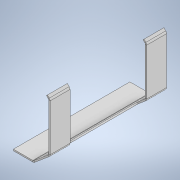
# Autodesk Inventor part: Trasera
Saved by Autodesk Inventor 2021 (Build 250183000, 183)
## iProperties
Created: 2021-07-21
Part Number: Trasera
Material: Generic
Document SubType Name: Sheet Metal
Designer: admin
Density: 1 g/cm^3
Sheet Metal Rule: Por defecto_mm
Appearance: Default
Flat Pattern Width: 32.5 cm
Flat Pattern Length: 41 cm
Flat Pattern Area: 1332.5 cm^2
Sheet Metal Width: 0.325 m
Sheet Metal Length: 0.410 m
Sheet Metal Area: 0.133 m^2
Author: admin
Autodesk Inventor part; units mm, degrees
ref_plane "YZ Plane" through (0, 0, 0) normal (1, 0, 0) x (0, 1, 0)
ref_plane "XZ Plane" through (0, 0, 0) normal (0, 1, 0) x (-1, 0, 0)
ref_plane "XY Plane" through (0, 0, 0) normal (0, 0, 1) x (1, 0, 0)
sketch "Boceto1" plane through (0, 0, 0) normal (0, 1, 0) x (-1, 0, 0)
  line L0 (162.5, 205) -> (-162.5, 205)
  line L1 (-162.5, -205) -> (162.5, -205)
  line L2 (162.5, -205) -> (162.5, 205)
  line L3 (162.5, 205) -> (-162.5, -205) construction
  line L4 (-162.5, 205) -> (162.5, -205) construction
  line L5 (-162.5, -205) -> (-162.5, -135)
  line L6 (-162.5, 205) -> (-162.5, 135)
  line L7 (-162.5, 0) -> (57.5, 0)
  line L8 (-162.5, 135) -> (57.5, 135)
  line L9 (57.5, 135) -> (57.5, -135)
  line L10 (57.5, -135) -> (-162.5, -135)
  line L11 (-162.5, 205) -> (-162.5, 135)
  line L12 (-162.5, -135) -> (-162.5, -205)
  point P0 (0, 0)
  dimension "d0" = 325
  dimension "d1" = 410
  dimension "d24" = 70
  dimension "d25" = 70
  dimension "d26" = 220
  constraints: 26 end point, 4 parallel, 2 horizontal, 2 midpoint, 2 perpendicular
  measures "d0" distance of L1.end L1.start
  measures "d1" distance of L1.start L0.end
  measures "d24" distance of L1.start L5.end
  measures "d25" distance of L6.end L0.end
  measures "d26" distance of L7.start L7.end
extrude "Placa1" add sketch "Boceto1" along normal blind 5
sketch "Boceto3" plane through (0, 5, 0) normal (0, 1, 0) x (1, 0, 0)
  line L0 (-162.5, 205) -> (162.5, 205) projected
  line L1 (-162.5, 205) -> (-91.5, 205)
  line L2 (-91.5, 205) -> (-19.5, 205)
  line L3 (-19.5, 205) -> (150.5, 205)
  line L4 (150.5, 205) -> (150.5, -205) construction
  line L5 (162.5, -205) -> (-162.5, -205) construction
  line L6 (-19.5, 205) -> (-19.5, -205) construction
  line L7 (-91.5, 205) -> (-91.5, -205) construction
  point P0 (0, 0)
  dimension "d27" = 71
  dimension "d28" = 72
  dimension "d29" = 170
  constraints: 12 end point, 5 point on line, 2 vertical, 1 perpendicular
  measures "d27" distance of L0.start L1.end
  measures "d28" distance of L1.end L2.end
  measures "d29" distance of L2.end L3.end
fold "Pliegue4" angle 45 bend radius 5 thickness 5 k factor 0.44 line from (150.5, 5, -205) to (150.5, 5, 205) line at bend centre moving side (1, 0, 0) folds toward (0, 1, 0)
fold "Pliegue5" angle 50 bend radius 5 thickness 5 k factor 0.44 line from (-19.5, 5, -205) to (-19.5, 5, 205) line at bend centre moving side (1, 0, 0) folds toward (0, 1, 0)
fold "Pliegue6" angle 40 bend radius 5 thickness 5 k factor 0.44 line from (-91.5, 5, -205) to (-91.5, 5, 205) line at bend centre moving side (1, 0, 0) folds toward (0, 1, 0)
equation "\"d2\" = Thickness"
equation "\"d30\" = BendReliefWidth"
equation "\"d31\" = BendReliefDepth"
equation "\"d32\" = MinimumRemnant"
equation "\"d33\" = TransitionRadius"
equation "\"d35\" = BendRadius"
equation "\"d36\" = BendReliefWidth"
equation "\"d37\" = BendReliefDepth"
equation "\"d38\" = MinimumRemnant"
equation "\"d39\" = TransitionRadius"
equation "\"d41\" = BendRadius"
equation "\"d42\" = BendReliefWidth"
equation "\"d43\" = BendReliefDepth"
equation "\"d44\" = MinimumRemnant"
equation "\"d45\" = TransitionRadius"
equation "\"d47\" = BendRadius"
equation "\"BendRadius\" = Thickness"
equation "\"BendReliefWidth\" = Thickness"
equation "\"BendReliefDepth\" = 0.5 * Thickness"
equation "\"TransitionRadius\" = BendRadius"
equation "\"JacobiRadiusSize\" = BendRadius"
equation "\"GapSize\" = Thickness"
equation "\"Thickness\" = 5"
equation "\"MinimumRemnant\" = 10"
